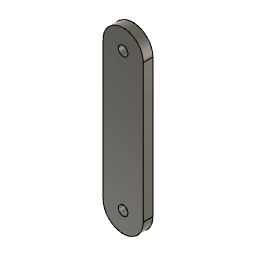
Crank_B v2 (Autodesk Fusion 360 design; units mm, degrees)
Autodesk Fusion 360 part; units mm, degrees
sketch "Sketch1" plane through (0, 0, 0) normal (0, 1, 0) x (1, 0, 0)
  arc A0 (12.5, 96.75) -> (-12.5, 96.75) centre (0, 96.75) ccw
  line L0 (12.5, 96.75) -> (12.5, 10.75)
  arc A1 (-12.5, 10.75) -> (12.5, 10.75) centre (0, 10.75) ccw
  circle A2 centre (0, 96.75) radius 3
  circle A3 centre (0, 10.75) radius 3
  line L1 (-12.5, 10.75) -> (-12.5, 96.75)
  constraint parallel L0 L1
  constraint concentric A1 A3
extrude "Extrude1" add sketch "Sketch1" along normal blind 6
